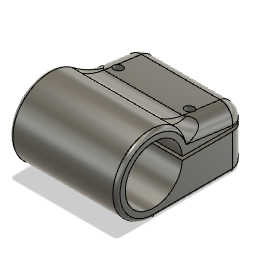
29part (Autodesk Fusion 360 design; units mm, degrees)
Autodesk Fusion 360 part; units mm, degrees
sketch "Sketch1" plane through (0, 0, 0) normal (1, 0, 0) x (0, 0, -1)
  circle A0 centre (0, 0) radius 16
  circle A1 centre (0, 0) radius 21
  line L0 (15.654332, 13.997925) -> (52, 9)
  line L1 (52, 9) -> (52, -21)
  line L2 (52, -21) -> (0, -21)
  line L3 (0, -21) -> (15.654332, 13.997925)
  line L4 (21, 8) -> (42, 8)
  line L5 (42, 8) -> (42, -21)
  line L6 (42, -21) -> (21, -21)
  line L7 (21, -21) -> (21, 8)
  line L8 (0, 1) -> (52, 1)
  line L9 (52, 1) -> (52, -1)
  line L10 (52, -1) -> (0, -1)
  line L11 (0, -1) -> (0, 1)
  dimension "d1" = 32
  dimension "d2" = 5
  dimension "d3" = 21
  dimension "d4" = 29
  dimension "d5" = 10
  dimension "d6" = 30
  dimension "d7" = 2
  constraint coincident A0.centre A1.centre
  constraint vertical L1
  constraint horizontal L2
  constraint coincident A1 L2.end
  constraint horizontal L4
  constraint vertical L5
  constraint horizontal L6
  constraint vertical L7
  constraint tangent A1 L7
  constraint collinear L2 L6
  constraint tangent A1 L2
  constraint tangent A0 L0
  constraint horizontal L8
  constraint vertical L9
  constraint horizontal L10
  constraint vertical L11
  constraint collinear L1 L9
  constraint midpoint A0.centre L11
  measures "d1" diameter of A0
  measures "d3" distance of L4.start L4.end
  measures "d4" distance of L4.start L6.end
  measures "d5" distance of L1 L5
  measures "d6" distance of L0.end L1.end
  measures "d7" distance of L8.end L9.end
extrude "Extrude1" add sketch "Sketch1" along normal blind 60 contours A0 A1 L3 L8 | A0 A1 L3 L10 | A0 A1 L3 | A1 L0 L1 L4 L5 L7 L8 | A1 L2 L7 L10 | L4 L5 L7 L8 | L2 L5 L6 L7 L10 | L1 L2 L5 L10 picked at (19.196767, 1.947608) picked at (19.194091, -1.961902) picked at (13.661076, 13.612607) picked at (48.666667, 6) picked at (16.637773, -17.108181) picked at (35, 5.666667) picked at (35, -14.333333) picked at (45.333333, -7.666667)
extrude "Extrude2" cut sketch "Sketch1" along normal mid plane 21 from surface at 30 contours L5 L7 L8 L10 | L4 L5 L7 L8 | L2 L5 L6 L7 L10 picked at (35, 0) picked at (35, 5.666667) picked at (35, -14.333333)
fillet "Fillet1" radius 2 4 edges at (60, 8.574485, 19.169721) (60, -21, -26) (0, 8.574485, 19.169721) (0, -21, -26)
fillet "Fillet2" radius 8 10 edges at (0, 11.727454, -32.165543) (0, 5, -52) (30, 9, -52) (0, -10, -52) (0.585786, -20.414214, -52) (30, -21, -52) (59.414214, -20.414214, -52) (60, -10, -52) (60, 5, -52) (60, 11.727454, -32.165543)
fillet "Fillet3" radius 30 5 edges at (0.551675, 8.473165, -18.534307) (4.570163, 13.115103, -16.40074) (30, 13.997925, -15.654332) (55.429837, 13.115103, -16.40074) (59.448325, 8.473165, -18.534307)
ref_plane "WorkPlane1" through (30, -22, -26) normal (0, -1, 0) x (0, 0, -1)
sketch "Sketch2" plane through (30, -22, -22) normal (0, -1, 0) x (1, 0, 0)
  circle A0 centre (-20, -8) radius 2.5
  circle A1 centre (20, -8) radius 2.5
  dimension "d17" = 5
  dimension "d20" = 40
  dimension "d21" = 0
  measures "d17" diameter of A0
extrude "Extrude3" cut sketch "Sketch2" against normal through all contours A0 | A1 picked at (-20.304451, -8.667648) picked at (19.695549, -8.667648)
